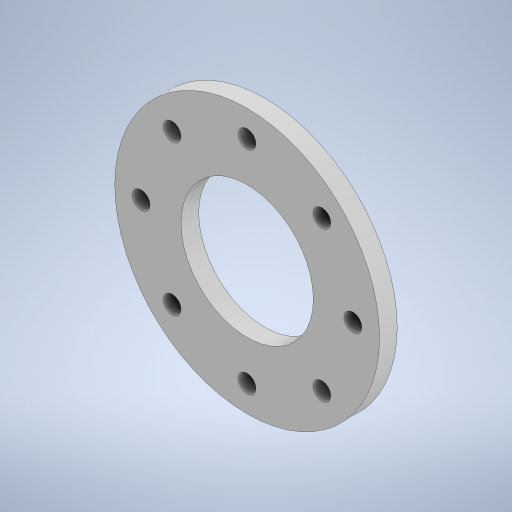
# Autodesk Inventor part: 05-22-2023 flangia
Saved by Autodesk Inventor 2023 (Build 270158000, 158)
## iProperties
Created: 2023-05-22
Part Number: 05-22-2023 flangia
Material: Generico
Document SubType Name: Modeling
Designer: Admin
Density: 1 g/cm^3
Appearance: Default
Author: Admin
Autodesk Inventor part; units mm, degrees
ref_plane "YZ Plane" through (0, 0, 0) normal (1, 0, 0) x (0, 1, 0)
ref_plane "XZ Plane" through (0, 0, 0) normal (0, 1, 0) x (-1, 0, 0)
ref_plane "XY Plane" through (0, 0, 0) normal (0, 0, 1) x (1, 0, 0)
sketch "Schizzo1" plane through (0, 0, 0) normal (0, 0, 1) x (1, 0, 0)
  circle A0 centre (0, 0) radius 150
  circle A1 centre (0, 0) radius 75
  circle A2 centre (-120, 0) radius 10
  circle A3 centre (-84.8528, 84.8528) radius 10
  circle A4 centre (0, 120) radius 10
  circle A5 centre (84.8528, 84.8528) radius 10
  circle A6 centre (120, 0) radius 10
  circle A7 centre (84.8528, -84.8528) radius 10
  circle A8 centre (0, -120) radius 10
  circle A9 centre (-84.8528, -84.8528) radius 10
  dimension "d0" = 150
  dimension "d1" = 300
  dimension "d2" = 20
  dimension "d5" = 360
  dimension "d9" = 120
  constraints: 10 centre point, 4 coincident, 1 horizontal alignment, 23 other
  measures "d0" diameter of A1
  measures "d1" diameter of A0
  measures "d2" diameter of A2
  measures "d9" distance of A0.centre A2.centre
extrude "Estrusione1" add sketch "Schizzo1" along normal mid plane 20
